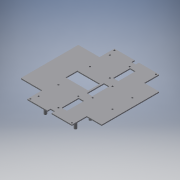
# Autodesk Inventor part: Part37
Saved by Autodesk Inventor 2016 (Build 200138000, 138)
## iProperties
Created: 2015-11-06
Part Number: Part37
Material: Generic
Document SubType Name: Modeling
Designer: Jufo
Density: 1 g/cm^3
Appearance: Default
Author: Jufo
Autodesk Inventor part; units mm, degrees
ref_plane "YZ Plane" through (0, 0, 0) normal (1, 0, 0) x (0, 1, 0)
ref_plane "XZ Plane" through (0, 0, 0) normal (0, 1, 0) x (-1, 0, 0)
ref_plane "XY Plane" through (0, 0, 0) normal (0, 0, 1) x (1, 0, 0)
sketch "Sketch3" plane through (0, 0, 0) normal (0, 1, 0) x (-1, 0, 0)
  line L0 (-63.7605, -81.8282) -> (-41.7605, -81.8282)
  line L1 (-41.7605, -81.8282) -> (-69.7605, -81.8282)
  line L2 (-41.7605, -81.8282) -> (-41.7605, -109.8282)
  line L3 (-41.7605, -81.8282) -> (-41.7605, -109.8282)
  line L4 (-41.7605, -109.8282) -> (-3.7605, -109.8282)
  line L5 (-3.7605, -109.8282) -> (-3.7605, -103.8282)
  line L6 (-3.7605, -109.8282) -> (-3.7605, -103.8282)
  line L7 (-3.7605, -103.8282) -> (4.2395, -103.8282)
  line L8 (4.2395, -103.8282) -> (4.2395, -109.8282)
  line L9 (4.2395, -109.8282) -> (42.2395, -109.8282)
  line L10 (42.2395, -109.8282) -> (42.2395, -81.8282)
  line L11 (42.2395, -109.8282) -> (42.2395, -81.8282)
  line L12 (42.2395, -81.8282) -> (82.2395, -81.8282)
  line L13 (82.2395, -81.8282) -> (82.2395, 26.1718)
  line L14 (42.2395, 26.1718) -> (66.2395, 26.1718)
  line L15 (82.2395, 26.1718) -> (42.2395, 26.1718)
  line L16 (42.2395, 26.1718) -> (42.2395, 54.1718)
  line L17 (42.2395, 54.1718) -> (4.2395, 54.1718)
  line L18 (4.2395, 48.1718) -> (-3.7605, 48.1718)
  line L19 (-3.7605, 48.1718) -> (-3.7605, 54.1718)
  line L20 (4.2395, 48.1718) -> (4.2395, 54.1718)
  line L21 (4.2395, 54.1718) -> (4.2395, 48.1718)
  line L22 (-3.7605, 54.1718) -> (-41.7605, 54.1718)
  line L23 (-41.7605, 54.1718) -> (-41.7605, 26.1718)
  line L24 (-41.7605, 54.1718) -> (-41.7605, 26.1718)
  line L25 (-41.7605, 26.1718) -> (-69.7605, 26.1718)
  line L26 (-69.7605, 26.1718) -> (-69.7605, -81.8282)
  point P0 (0, 0)
  dimension "d1" = 108
  dimension "d2" = 108
  dimension "d3" = 164
  dimension "d4" = 164
  dimension "d6" = 28
  dimension "d7" = 28
  dimension "d11" = 28
  dimension "d12" = 38
  dimension "d13" = 38
  dimension "d14" = 38
  dimension "d15" = 38
  dimension "d16" = 40
  dimension "d18" = 8
  dimension "d19" = 8
  dimension "d21" = 28
  constraints: 54 end point, 9 perpendicular, 6 collinear, 3 horizontal
  measures "d1" distance of L25.end L1.end
  measures "d2" distance of L12.end L13.end
  measures "d3" distance of L22.end L2.end
  measures "d4" distance of L9.end L16.end
  measures "d6" distance of L9.end L10.end
  measures "d7" distance of L0.end L2.end
  measures "d11" distance of L14.start L16.end
  measures "d12" distance between parallel lines of L16 L20
  measures "d13" distance between parallel lines of L23 L19
  measures "d14" distance from line of L7.end L10
  measures "d15" distance from line of L2 L5.end
  measures "d16" distance of L13.end L14.start
  measures "d18" distance of L18.start L18.end
  measures "d19" distance of L5.end L7.end
  measures "d21" distance of L0.end L1.end
extrude "Extrusion1" add sketch "Sketch3" along normal blind 2
sketch "Sketch7" plane through (0, 0, 0) normal (0, -1, 0) x (1, 0, 0)
  circle A0 centre (34.1141, 39.7322) radius 1.5
  circle A1 centre (34.1141, 11.8049) radius 1.5
  line L0 (34.1141, 39.7322) -> (34.1141, 11.8049)
  circle A2 centre (-16.6732, -3.4351) radius 1.5
  line L1 (34.1141, 11.8049) -> (-16.6732, -3.4351)
  circle A3 centre (-17.8162, 44.482) radius 1.5
  line L2 (-16.6732, -3.4351) -> (-17.8162, 44.482)
  line L3 (-17.8162, 44.482) -> (34.1141, 39.7322)
  circle A4 centre (34.1141, 39.7322) radius 2.5
  circle A5 centre (-17.8162, 44.482) radius 2.5
  circle A6 centre (-16.6732, -3.4351) radius 2.5
  circle A7 centre (34.1141, 11.8049) radius 2.5
  point P0 (0, 0)
  point P1 (-0.254, 0)
  dimension "d24" = 51.9303
  dimension "d25" = 27.9273
  dimension "d26" = 50.7873
  dimension "d27" = 47.9171
  dimension "d28" = 5
  dimension "d29" = 3
  dimension "d30" = 3
  dimension "d31" = 3
  dimension "d32" = 3
  dimension "d33" = 5
  dimension "d34" = 5
  dimension "d35" = 5
  constraints: 8 centre point, 8 end point, 4 coincident, 1 vertical
  measures "d24" horizontal distance of L2.end L0.start
  measures "d25" distance of L0.start L0.end
  measures "d26" horizontal distance of L0.end L1.end
  measures "d27" vertical distance of L1.end L2.end
  measures "d28" diameter of A4
  measures "d29" diameter of A0
  measures "d30" diameter of A1
  measures "d31" diameter of A2
  measures "d32" diameter of A3
  measures "d33" diameter of A5
  measures "d34" diameter of A6
  measures "d35" diameter of A7
extrude "Extrusion2" add sketch "Sketch7" along normal blind 15 contours A0 L3 A4 L0 | A0 L0 A4 L3 | A5 L2 A3 L3 | L3 A3 L2 A5 | A7 L1 A1 L0 | L0 A1 L1 A7 | A6 L1 A2 L2 | L2 A2 L1 A6
sketch "Sketch8" plane through (0, 0, 0) normal (0, -1, 0) x (1, 0, 0)
  circle A0 centre (-17.7942, -100.0771) radius 1.5
  circle A1 centre (-16.6512, -52.16) radius 1.5
  line L0 (-17.7942, -100.0771) -> (-16.6512, -52.16)
  circle A2 centre (34.1361, -67.4) radius 1.5
  line L1 (-16.6512, -52.16) -> (34.1361, -67.4)
  circle A3 centre (34.1361, -95.3273) radius 1.5
  line L2 (34.1361, -67.4) -> (34.1361, -95.3273)
  line L3 (34.1361, -95.3273) -> (-17.7942, -100.0771)
  circle A4 centre (34.1361, -95.3273) radius 2.5
  circle A5 centre (34.1361, -67.4) radius 2.5
  circle A6 centre (-16.6512, -52.16) radius 2.5
  circle A7 centre (-17.7942, -100.0771) radius 2.5
  point P0 (0, 0)
  point P1 (-0.254, 0)
  dimension "d38" = 47.9171
  dimension "d39" = 51.9303
  dimension "d40" = 27.9273
  dimension "d41" = 50.7873
  dimension "d42" = 32.6771
  dimension "d43" = 43.1673
  dimension "d44" = 50.7873
  dimension "d45" = 3
  dimension "d46" = 3
  dimension "d47" = 3
  dimension "d48" = 3
  dimension "d49" = 5
  dimension "d50" = 5
  dimension "d51" = 5
  dimension "d52" = 5
  constraints: 8 centre point, 8 end point, 4 coincident, 1 vertical
  measures "d38" vertical distance of L0.start L0.end
  measures "d39" horizontal distance of L2.end L0.start
  measures "d40" distance of L1.end L2.end
  measures "d41" horizontal distance of L0.end L1.end
  measures "d42" vertical distance of L1.end L0.start
  measures "d43" vertical distance of L2.end L0.end
  measures "d44" horizontal distance of L2.end L0.end
  measures "d45" diameter of A0
  measures "d46" diameter of A1
  measures "d47" diameter of A2
  measures "d48" diameter of A3
  measures "d49" diameter of A4
  measures "d50" diameter of A5
  measures "d51" diameter of A6
  measures "d52" diameter of A7
extrude "Extrusion3" add sketch "Sketch8" along normal blind 5 contours A0 L3 A7 L0 | A0 L0 A7 L3 | A4 L2 A3 L3 | L3 A3 L2 A4 | A6 L1 A1 L0 | L0 A1 L1 A6 | A5 L1 A2 L2 | L2 A2 L1 A5
sketch "Sketch9" plane through (0, 2, 0) normal (0, 1, 0) x (1, 0, 0)
  circle A0 centre (38.7605, 106.8282) radius 1.5
  line L0 (41.7605, 109.8282) -> (3.7605, 109.8282) projected
  line L1 (41.7605, 81.8282) -> (41.7605, 109.8282) projected
  line L2 (69.7605, -26.1718) -> (69.7605, 81.8282) projected
  line L3 (69.7605, 27.8282) -> (-19.2089, 27.8282)
  line L4 (-0.2395, 109.8282) -> (-0.2395, 42.6367)
  circle A1 centre (-39.2395, 106.8282) radius 1.5
  circle A2 centre (38.7605, -51.1718) radius 1.5
  circle A3 centre (-39.2395, -51.1718) radius 1.5
  point P0 (0, 0)
  dimension "d55" = 3
  dimension "d56" = 3
  dimension "d57" = 3
  constraints: 4 centre point, 4 end point, 3 symmetric about line, 1 horizontal, 1 midpoint, 1 point on line, 1 vertical, 3 other
  measures "d55" diameter of A0
  measures "d56" distance from line of L0 A0.centre
  measures "d57" distance from line of L1 A0.centre
extrude "Extrusion4" cut sketch "Sketch9" against normal blind 10
sketch "Sketch10" plane through (0, 2, 0) normal (0, 1, 0) x (1, 0, 0)
  circle A0 centre (-35.8395, -39.1718) radius 1.5
  circle A1 centre (-35.8395, -39.1718) radius 1.5
  circle A2 centre (-35.8395, -1.8718) radius 1.5
  circle A3 centre (-35.8395, -1.8718) radius 1.5
  circle A4 centre (1.4605, -1.8718) radius 1.5
  circle A5 centre (1.4605, -1.8718) radius 1.5
  circle A6 centre (1.4605, -39.1718) radius 1.5
  circle A7 centre (1.4605, -39.1718) radius 1.5
  line L0 (-42.2395, -54.1718) -> (-4.2395, -54.1718) projected
  line L1 (-42.2395, -26.1718) -> (-42.2395, -54.1718) projected
  line L2 (3.7605, -54.1718) -> (41.7605, -54.1718) projected
  point P0 (0, 0)
  point P1 (22.3, 43.3)
  dimension "d60" = 37.3
  dimension "d61" = 37.3
  dimension "d62" = 37.3
  dimension "d63" = 37.3
  dimension "d64" = 15
  dimension "d65" = 6.4
  dimension "d66" = 6.4
  dimension "d67" = 15
  constraints: 8 centre point, 4 coincident
  measures "d60" distance of A7.centre A5.centre
  measures "d61" distance of A1.centre A7.centre
  measures "d62" distance of A3.centre A5.centre
  measures "d63" distance of A3.centre A1.centre
  measures "d64" distance from line of L0 A1.centre
  measures "d65" distance from line of L1 A0.centre
  measures "d66" distance from line of L1 A2.centre
  measures "d67" distance from line of L2 A6.centre
extrude "Extrusion5" cut sketch "Sketch10" against normal blind 10
sketch "Sketch11" plane through (0, 2, 0) normal (0, 1, 0) x (1, 0, 0)
  circle A0 centre (-35.8395, 57.5282) radius 1.5
  circle A1 centre (-35.8395, 57.5282) radius 1.5
  circle A2 centre (-35.8395, 94.8282) radius 1.5
  circle A3 centre (-35.8395, 94.8282) radius 1.5
  circle A4 centre (1.4605, 94.8282) radius 1.5
  circle A5 centre (1.4605, 94.8282) radius 1.5
  circle A6 centre (1.4605, 57.5282) radius 1.5
  circle A7 centre (1.4605, 57.5282) radius 1.5
  line L0 (-4.2395, 109.8282) -> (-42.2395, 109.8282) projected
  line L1 (-42.2395, 109.8282) -> (-42.2395, 81.8282) projected
  point P0 (0, 0)
  point P1 (22.3, 43.3)
  dimension "d70" = 37.3
  dimension "d71" = 37.3
  dimension "d72" = 37.3
  dimension "d73" = 37.3
  dimension "d74" = 15
  dimension "d75" = 15
  dimension "d105" = 6.4
  dimension "d106" = 6.4
  constraints: 8 centre point, 4 coincident
  measures "d70" distance of A7.centre A5.centre
  measures "d71" distance of A1.centre A7.centre
  measures "d72" distance of A3.centre A1.centre
  measures "d73" distance of A3.centre A5.centre
  measures "d74" distance from line of L0 A4.centre
  measures "d75" distance from line of L0 A2.centre
  measures "d105" distance from line of L1 A3.centre
  measures "d106" distance from line of L1 A1.centre
extrude "Extrusion6" cut sketch "Sketch11" against normal blind 10
sketch "Sketch12" plane through (0, 2, 0) normal (0, 1, 0) x (1, 0, 0)
  circle A0 centre (17.4605, 9.1782) radius 1.5
  circle A1 centre (17.4605, 9.1782) radius 1.5
  circle A2 centre (17.4605, 46.4782) radius 1.5
  circle A3 centre (17.4605, 46.4782) radius 1.5
  circle A4 centre (54.7605, 46.4782) radius 1.5
  circle A5 centre (54.7605, 46.4782) radius 1.5
  circle A6 centre (54.7605, 9.1782) radius 1.5
  circle A7 centre (54.7605, 9.1782) radius 1.5
  line L0 (69.7605, -26.1718) -> (69.7605, 81.8282) projected
  line L1 (41.7605, -26.1718) -> (69.7605, -26.1718) projected
  point P0 (0, 0)
  point P1 (22.3, 43.3)
  dimension "d80" = 37.3
  dimension "d81" = 37.3
  dimension "d82" = 37.3
  dimension "d83" = 37.3
  dimension "d84" = 15
  dimension "d85" = 15
  dimension "d86" = 35.35
  dimension "d87" = 35.35
  constraints: 8 centre point, 4 coincident
  measures "d80" distance of A4.centre A6.centre
  measures "d81" distance of A1.centre A7.centre
  measures "d82" distance of A3.centre A1.centre
  measures "d83" distance of A5.centre A3.centre
  measures "d84" distance from line of L0 A4.centre
  measures "d85" distance from line of L0 A6.centre
  measures "d86" distance from line of L1 A6.centre
  measures "d87" distance from line of L1 A0.centre
extrude "Extrusion7" cut sketch "Sketch12" against normal blind 10
sketch "Sketch13" plane through (0, 2, 0) normal (0, 1, 0) x (1, 0, 0)
  line L0 (14.4605, 43.4782) -> (4.4605, 43.4782)
  line L1 (4.4605, 43.4782) -> (4.4605, 11.4782)
  line L2 (4.4605, 11.4782) -> (14.4605, 11.4782)
  line L3 (14.4605, 11.4782) -> (14.4605, 43.4782)
  circle A0 centre (17.4605, 46.4782) radius 1.5 projected
  line L4 (4.4605, 60.5282) -> (14.4605, 60.5282)
  line L5 (14.4605, 60.5282) -> (14.4605, 92.5282)
  line L6 (14.4605, 92.5282) -> (4.4605, 92.5282)
  line L7 (4.4605, 92.5282) -> (4.4605, 60.5282)
  circle A1 centre (1.4605, 57.5282) radius 1.5 projected
  line L8 (4.4605, -36.1718) -> (14.4605, -36.1718)
  line L9 (14.4605, -36.1718) -> (14.4605, -4.1718)
  line L10 (14.4605, -4.1718) -> (4.4605, -4.1718)
  line L11 (4.4605, -4.1718) -> (4.4605, -36.1718)
  circle A2 centre (1.4605, -39.1718) radius 1.5 projected
  point P0 (0, 0)
  dimension "d60" = 37.3
  dimension "d90" = 10
  dimension "d91" = 32
  dimension "d92" = 3
  dimension "d93" = 32
  dimension "d94" = 10
  dimension "d95" = 3
  dimension "d97" = 3
  dimension "d98" = 3
  dimension "d99" = 32
  dimension "d100" = 3
  dimension "d101" = 3
  dimension "d102" = 10
  constraints: 24 end point, 6 parallel, 3 horizontal, 3 perpendicular
  measures "d90" distance of L2.end L1.end
  measures "d91" distance of L1.end L0.end
  measures "d92" distance from line of A0.centre L0
  measures "d93" distance of L4.end L5.end
  measures "d94" distance of L5.end L6.end
  measures "d95" distance from line of L4 A1.centre
  measures "d97" distance from line of A0.centre L3
  measures "d98" distance from line of L7 A1.centre
  measures "d99" distance of L9.end L8.end
  measures "d100" distance from line of L8 A2.centre
  measures "d101" distance from line of L11 A2.centre
  measures "d102" distance of L9.end L10.end
extrude "Extrusion8" cut sketch "Sketch13" against normal blind 10 contours L3 L2 L1 L0 | L7 L6 L5 L4 | L11 L10 L9 L8
sketch "Sketch14" plane through (0, 2, 0) normal (0, 1, 0) x (1, 0, 0)
  line L0 (-41.0232, 16.8213) -> (-41.0232, 38.8213)
  line L1 (-41.0232, 38.8213) -> (1.4768, 38.8213)
  line L2 (1.4768, 38.8213) -> (1.4768, 16.8213)
  line L3 (1.4768, 16.8213) -> (-41.0232, 16.8213)
  point P0 (0, 0)
  dimension "d107" = 22
  dimension "d108" = 42.5
  constraints: 8 end point, 3 perpendicular, 1 vertical
  measures "d107" distance of L0.start L0.end
  measures "d108" distance of L0.end L1.end
extrude "Extrusion9" cut sketch "Sketch14" against normal blind 10
equation "\"d7\" = d6"
equation "\"d12\" = d13"
equation "\"d14\" = d13"
equation "\"d15\" = d13"
equation "\"d66\" = d65"
equation "\"d67\" = d64"
equation "\"d75\" = d74"
equation "\"d106\" = d105"
equation "\"d85\" = d84"
equation "\"d87\" = d86"
body "Solid1"
